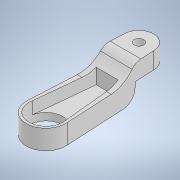
# Autodesk Inventor part: Поворотный рычаг для сервы
Saved by Autodesk Inventor 2020 (Build 240168000, 168)
## iProperties
Created: 2021-04-11
Part Number: Поворотный рычаг для сервы
Material: Типовые
Document SubType Name: Modeling
Designer: Антон
Density: 1 g/cm^3
Appearance: По умолчанию
Длина_рычага: 19,000 мм
Author: Антон
Autodesk Inventor part; units mm, degrees
ref_plane "YZ Plane" through (0, 0, 0) normal (1, 0, 0) x (0, 1, 0)
ref_plane "XZ Plane" through (0, 0, 0) normal (0, 1, 0) x (-1, 0, 0)
ref_plane "XY Plane" through (0, 0, 0) normal (0, 0, 1) x (1, 0, 0)
sketch "Эскиз1" plane through (0, 0, 0) normal (0, 1, 0) x (-1, 0, 0)
  circle A0 centre (0, 0) radius 4
  dimension "d0" = 8
  constraints: 1 centre point, 1 coincident
  measures "d0" diameter of A0
extrude "Выдавливание1" add sketch "Эскиз1" along normal blind 4
sketch "Эскиз5" plane through (0, 4, 0) normal (0, 1, 0) x (1, 0, 0)
  circle A0 centre (0, 0) radius 4 projected
  line L0 (-4, 0) -> (4, 0)
  line L1 (4, 0) -> (4, 19)
  line L2 (4, 19) -> (-4, 19)
  line L3 (-4, 19) -> (-4, 0)
  circle A1 centre (0, 0) radius 4 projected
  circle A2 centre (0, 19) radius 3
  line L4 (4, 0) -> (3, 19)
  line L5 (-4, 0) -> (-3, 19)
  point P0 (4, 0)
  point P1 (-3.9779, 0.4199)
  point P2 (3.9779, 0.4199)
  dimension "Длина_рычага" = 19
  dimension "d59" = 6
  constraints: 12 end point, 3 point on circle, 2 midpoint, 2 parallel, 2 point on line, 1 centre point, 1 coincident, 1 horizontal, 1 perpendicular, 2 other
  measures "Длина_рычага" distance of L1.end L0.end
  measures "d59" diameter of A2
extrude "Выдавливание4" add sketch "Эскиз5" against normal blind 4 contours A0 L5 A2 L4 | A2 L2 | L2 A2
sketch "Эскиз9" plane through (0, 4, 0) normal (0, -1, 0) x (1, 0, 0)
  circle A0 centre (0, 0) radius 3.5
  line L0 (3.5, 0) -> (-3.5, 0)
  line L1 (3.5, 0) -> (2.25, -12.5)
  line L2 (-3.5, 0) -> (-2.25, -12.5)
  line L3 (2.25, -12.5) -> (-2.25, -12.5)
  point P0 (0, -12.5)
  point P1 (-3.4307, -0.6931)
  point P2 (3.4307, -0.6931)
  dimension "d43" = 7
  dimension "d44" = 4.5
  dimension "d45" = 12.5
  constraints: 8 end point, 2 coincident, 2 horizontal, 2 midpoint, 2 point on circle, 1 centre point, 1 equal length, 1 vertical alignment
  measures "d43" diameter of A0
  measures "d44" distance of L1.end L2.end
  measures "d45" distance from line of L3 point (0, 0)
extrude "Выдавливание7" cut sketch "Эскиз9" along normal blind 2.5
sketch "Эскиз10" plane through (0, 1.5, 0) normal (0, 1, 0) x (1, 0, 0)
  line L0 (2.25, 12.5) -> (3.4307, 0.6931) projected
  line L1 (-3.4307, 0.6931) -> (-2.25, 12.5) projected
  arc A0 (-3.4307, 0.6931) -> (3.4307, 0.6931) centre (0, 0) ccw projected
  arc A1 (-3.4307, 0.6931) -> (3.4307, 0.6931) centre (0, 0) ccw projected
  circle A2 centre (0, 0) radius 3.5
  line L2 (-2.25, 12.5) -> (2.25, 12.5) projected
  point P0 (3.4307, 0.6931)
  constraints: 1 coincident, 3 other
extrude "Выдавливание8" cut sketch "Эскиз10" against normal through all contours A0 A2
sketch "Эскиз13" plane through (0, 0, 0) normal (0, -1, 0) x (1, 0, 0)
  arc A0 (-3, -19) -> (3, -19) centre (0, -19) ccw projected
  circle A1 centre (0, -19) radius 3
  line L0 (-2.25, -12.5) -> (2.25, -12.5) projected
  line L1 (-2.25, -12.5) -> (2.25, -12.5) projected
  line L2 (3.2105, -15) -> (-3.2105, -15)
  line L3 (-3.2105, -15) -> (-3.2105, -22)
  line L4 (-3.2105, -22) -> (3.2105, -22)
  line L5 (3.2105, -22) -> (3.2105, -15)
  line L6 (-3.9779, -0.4199) -> (-3, -19) projected
  line L7 (3, -19) -> (3.9779, -0.4199) projected
  point P0 (0, 0)
  point P1 (3, -19)
  point P2 (-3, -19)
  dimension "d71" = 7
  constraints: 8 end point, 2 parallel, 2 point on line, 2 tangent, 1 centre point, 1 coincident, 1 horizontal, 1 perpendicular
  measures "d71" distance of L4.end L2.start
extrude "Выдавливание10" cut sketch "Эскиз13" against normal blind 3.5 contours A1 A0 | L6 L2 L7 A1
sketch "Эскиз14" plane through (0, 3.5, -19) normal (0, -1, 0) x (-1, 0, 0)
  arc A0 (3, 0) -> (-3, 0) centre (0, 0) ccw projected
  line L0 (-3.2105, -4) -> (-3, 0) projected
  line L1 (3, 0) -> (3.2105, -4) projected
  line L2 (3.2105, -4) -> (-3.2105, -4) projected
  point P0 (0, -19)
hole "Отверстие4" at (0, 3.5, -19) direction (0, 1, 0) diameter 1.95 depth 4
sketch "Эскиз15" plane through (0, 4, 0) normal (0, 1, 0) x (1, 0, 0)
  circle A0 centre (0, 19) radius 0.975 projected
  arc A1 (3, 19) -> (-3, 19) centre (0, 19) ccw projected
  line L0 (3.2105, 15) -> (3, 19) projected
  line L1 (-3, 19) -> (-3.2105, 15) projected
  line L2 (-3.2105, 15) -> (3.2105, 15) projected
  point P0 (0, 0)
extrude "Выдавливание11" add sketch "Эскиз15" along normal blind 2.9
fillet "Сопряжение1" radius 6 1 edges at (0, 4, -15)
fillet "Сопряжение1" radius 2.5 2 edges at (0, 6.9, -15) (0, 0, -15)
